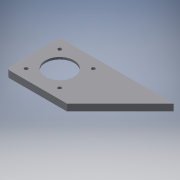
# Autodesk Inventor part: SUPORTE_MOTOR_EIXO_Y_1
Saved by Autodesk Inventor 2018 (Build 220112000, 112)
## iProperties
Created: 2018-10-11
Part Number: SUPORTE_MOTOR_EIXO_Y_1
Material: Genérico
Document SubType Name: Modeling
Designer: Usuario
Density: 1 g/cm^3
Appearance: Padrão
Author: Usuario
Autodesk Inventor part; units mm, degrees
ref_plane "YZ Plane" through (0, 0, 0) normal (1, 0, 0) x (0, 1, 0)
ref_plane "XZ Plane" through (0, 0, 0) normal (0, 1, 0) x (-1, 0, 0)
ref_plane "XY Plane" through (0, 0, 0) normal (0, 0, 1) x (1, 0, 0)
sketch "Esboço1" plane through (0, 0, 0) normal (0, 0, 1) x (1, 0, 0)
  line L0 (-33, -50) -> (-33, 950) projected
  line L1 (47, -50) -> (47, 950) projected
  line L2 (-73, -89.8276) -> (47, -89.8276)
  line L3 (47, -9.8276) -> (-73, -9.8276)
  line L4 (-73, -9.8276) -> (-73, -89.8276)
  line L5 (47, -89.8276) -> (47, -9.8276)
  point P0 (0, 0)
  dimension "d0" = 120
  dimension "d1" = 120
  dimension "d2" = 80
  constraints: 8 end point, 1 collinear, 1 horizontal, 1 parallel, 1 point on line
  measures "d0" distance of L3.start L3.end
  measures "d1" distance of L2.start L2.end
  measures "d2" distance of L3.end L2.start
extrude "Extrusão1" add sketch "Esboço1" along normal blind 9.52
sketch "Esboço9" plane through (0, 0, 0) normal (0, 0, -1) x (-1, 0, 0)
  line L0 (65, -22.8276) -> (6, -22.8276)
  line L1 (6, -22.8276) -> (6, -81.8276)
  line L2 (6, -81.8276) -> (65, -81.8276)
  line L3 (65, -81.8276) -> (65, -22.8276)
  line L4 (65, -22.8276) -> (6, -81.8276) construction
  line L5 (6, -22.8276) -> (65, -81.8276) construction
  line L6 (65, -52.3276) -> (6, -52.3276) construction
  line L7 (35.5, -22.8276) -> (35.5, -81.8276) construction
  circle A0 centre (59.07, -28.7576) radius 2.5
  circle A1 centre (59.07, -75.8976) radius 2.5
  circle A2 centre (11.93, -28.7576) radius 2.5
  circle A3 centre (11.93, -75.8976) radius 2.5
  line L8 (73, -9.8276) -> (73, -89.8276) projected
  line L9 (73, -89.8276) -> (-47, -89.8276) projected
  circle A4 centre (35.5, -52.3276) radius 20
  point P0 (0, 0)
  dimension "d72" = 59
  dimension "d73" = 59
  dimension "d74" = 5
  dimension "d75" = 5
  dimension "d76" = 5
  dimension "d77" = 5
  dimension "d78" = 23.57
  dimension "d79" = 23.57
  dimension "d80" = 23.57
  dimension "d81" = 23.57
  dimension "d82" = 23.57
  dimension "d83" = 23.57
  dimension "d84" = 23.57
  dimension "d85" = 23.57
  dimension "d86" = 8
  dimension "d87" = 8
  dimension "d88" = 40
  constraints: 16 end point, 5 centre point, 5 midpoint, 2 parallel, 1 horizontal, 1 perpendicular
  measures "d72" distance of L2.end L1.end
  measures "d73" distance of L1.end L0.end
  measures "d74" diameter of A0
  measures "d75" diameter of A1
  measures "d76" diameter of A2
  measures "d77" diameter of A3
  measures "d78" distance from line of L6 A3.centre
  measures "d79" distance from line of L7 A3.centre
  measures "d80" distance from line of L7 A1.centre
  measures "d81" distance from line of L6 A1.centre
  measures "d82" distance from line of L6 A0.centre
  measures "d83" distance from line of L7 A0.centre
  measures "d84" distance from line of L7 A2.centre
  measures "d85" distance from line of L6 A2.centre
  measures "d86" distance between parallel lines of L8 L3
  measures "d87" distance between parallel lines of L9 L2
  measures "d88" diameter of A4
extrude "Extrusão6" cut sketch "Esboço9" against normal blind 6.52
sketch "Esboço10" plane through (-35.5, -52.3276, 0) normal (0, 0, -1) x (-1, 0, 0)
  circle A0 centre (0, 0) radius 20 projected
  circle A1 centre (0, 0) radius 20
  circle A2 centre (23.57, -23.57) radius 2.5 projected
  circle A3 centre (23.57, -23.57) radius 2.5
  circle A4 centre (23.57, 23.57) radius 2.5 projected
  circle A5 centre (23.57, 23.57) radius 2.5
  circle A6 centre (-23.57, 23.57) radius 2.5 projected
  circle A7 centre (-23.57, 23.57) radius 2.5
  circle A8 centre (-23.57, -23.57) radius 2.5 projected
  circle A9 centre (-23.57, -23.57) radius 2.5
  point P0 (-35.5, 52.3276)
  constraints: 5 centre point, 5 coincident
extrude "Extrusão7" cut sketch "Esboço10" against normal through all
fillet "Arredondamento1" radius 6 4 edges at (-65, -22.8276, 3.26) (-65, -81.8276, 3.26) (-6, -22.8276, 3.26) (-6, -81.8276, 3.26)
fillet "Arredondamento2" radius 5 2 edges at (-73, -9.8276, 4.76) (-73, -89.8276, 4.76)
equation "\"d0\" = d1"
equation "\"d79\" = d78"
equation "\"d80\" = d78"
equation "\"d81\" = d78"
equation "\"d82\" = d78"
equation "\"d83\" = d78"
equation "\"d84\" = d78"
equation "\"d85\" = d78"
